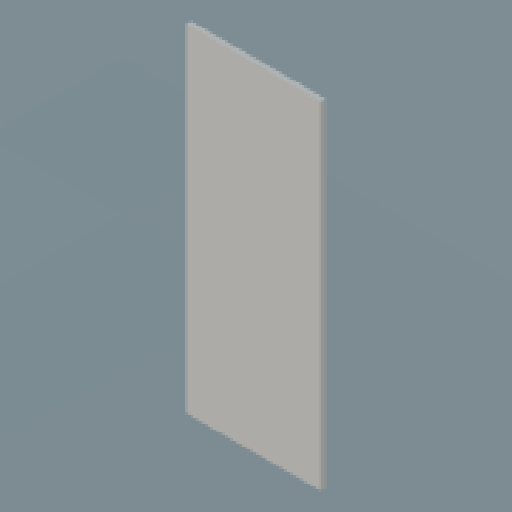
# Autodesk Inventor part: Drag Chain Guide Z Axis
Saved by Autodesk Inventor 2023.2 (Build 272271000, 271)
## iProperties
Created: 2023-02-19
Part Number: Drag Chain Guide Z Axis
Material: Aluminum 6061
Document SubType Name: Modeling
Designer: remop
Density: 2.7 g/cm^3
Appearance: Aluminum - Flat
Author: remop
Autodesk Inventor part; units mm, degrees
ref_plane "YZ Plane" through (0, 0, 0) normal (1, 0, 0) x (0, 1, 0)
ref_plane "XZ Plane" through (0, 0, 0) normal (0, 1, 0) x (-1, 0, 0)
ref_plane "XY Plane" through (0, 0, 0) normal (0, 0, 1) x (1, 0, 0)
sketch "Sketch1" plane through (0, 0, 0) normal (0, 0, 1) x (1, 0, 0)
  line L0 (-40, 100) -> (40, 100)
  line L1 (40, 100) -> (40, -100)
  line L2 (40, -100) -> (-40, -100)
  line L3 (-40, -100) -> (-40, 100)
  line L4 (-40, 100) -> (40, -100) construction
  line L5 (40, 100) -> (-40, -100) construction
  point P0 (0, 0)
  dimension "d0" = 80
  dimension "d1" = 200
  constraints: 12 end point, 2 midpoint, 2 parallel, 1 horizontal, 1 perpendicular
  measures "d0" distance of L1.end L2.end
  measures "d1" distance of L0.end L1.end
extrude "Extrusion1" add sketch "Sketch1" along normal blind 3
sketch "Sketch2" plane through (0, 0, 0) normal (0, 0, -1) x (-1, 0, 0)
  line L0 (40, -100) -> (-40, -100) projected
  line L1 (40, 100) -> (40, -100) projected
  line L2 (-40, 100) -> (40, 100) projected
  line L3 (-40, -100) -> (-40, 100) projected
  point P0 (0, 0)
  point P1 (32.5, -60)
  point P2 (32.5, 60)
  dimension "d4" = 7.5
  dimension "d5" = 7.5
  dimension "d6" = 40
  dimension "d7" = 40
  measures "d4" distance from line of L1 point (32.5, 60)
  measures "d5" distance from line of L1 point (32.5, -60)
  measures "d6" distance from line of L0 point (32.5, -60)
  measures "d7" distance from line of L2 point (32.5, 60)
hole "Hole1" at (-32.5, -60, 0) at (-32.5, 60, 0) direction (0, 0, 1) diameter 3.5 end through all
fillet "Fillet1" radius 3 4 edges at (-40, -100, 1.5) (40, -100, 1.5) (40, 100, 1.5) (-40, 100, 1.5)
sketch "Sketch3" plane through (0, 0, 0) normal (0, 0, -1) x (-1, 0, 0)
  arc A0 (40, 97) -> (37, 100) centre (37, 97) ccw projected
  line L0 (-37, 100) -> (37, 100) projected
  arc A1 (-37, 100) -> (-40, 97) centre (-37, 97) ccw projected
  line L1 (-40, -97) -> (-40, 97) projected
  arc A2 (-40, -97) -> (-37, -100) centre (-37, -97) ccw projected
  line L2 (37, -100) -> (-37, -100) projected
  arc A3 (37, -100) -> (40, -97) centre (37, -97) ccw projected
  line L3 (40, 97) -> (40, -97) projected
  circle A4 centre (32.5, -60) radius 1.75 projected
  circle A5 centre (32.5, 60) radius 1.75 projected
  line L4 (0, -85) -> (25, -85)
  line L5 (25, -85) -> (25, -38.3333)
  line L6 (25, -38.3333) -> (0, -38.3333)
  line L7 (0, -38.3333) -> (0, -85)
  line L8 (25, 85) -> (0, 85)
  line L9 (0, 85) -> (0, 38.3333)
  line L10 (0, 38.3333) -> (25, 38.3333)
  line L11 (25, 38.3333) -> (25, 85)
  line L12 (25, -23.3333) -> (0, -23.3333)
  line L13 (0, -23.3333) -> (0, 23.3333)
  line L14 (0, 23.3333) -> (25, 23.3333)
  line L15 (25, 23.3333) -> (25, -23.3333)
  point P0 (0, 0)
  point P1 (12.5, -23.3333)
  dimension "d16" = 15
  dimension "d17" = 15
  dimension "d18" = 15
  dimension "d19" = 15
  dimension "d20" = 15
  dimension "d21" = 25
  constraints: 24 end point, 6 parallel, 3 equal length, 3 horizontal, 3 perpendicular, 3 point on line, 1 midpoint
  measures "d16" distance from line of point (12.5, -23.333) L6
  measures "d17" distance between parallel lines of L10 L14
  measures "d18" distance between parallel lines of L0 L8
  measures "d19" distance between parallel lines of L2 L4
  measures "d20" distance between parallel lines of L3 L5
  measures "d21" distance of L4.start L4.end
extrude "Extrusion2" cut sketch "Sketch3" against normal through all contours L7 L6 L5 L4 | L11 L10 L9 L8 | L12 L13 L14 L15
equation "\"d5\" = d4"
equation "\"d7\" = d6"
equation "\"d17\" = d16"
equation "\"d18\" = d16"
equation "\"d19\" = d16"
body "Solid1"
